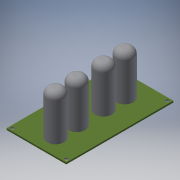
# Autodesk Inventor part: PCB
Saved by Autodesk Inventor 2017 (Build 210142000, 142)
## iProperties
Created: 2018-01-14
Part Number: PCB
Material: Generic
Document SubType Name: Modeling
Designer: Mitch
Density: 1 g/cm^3
Appearance: Default
Author: Mitch
Autodesk Inventor part; units mm, degrees
ref_plane "YZ Plane" through (0, 0, 0) normal (1, 0, 0) x (0, 1, 0)
ref_plane "XZ Plane" through (0, 0, 0) normal (0, 1, 0) x (-1, 0, 0)
ref_plane "XY Plane" through (0, 0, 0) normal (0, 0, 1) x (1, 0, 0)
sketch "Sketch3" plane through (0, 0, 0) normal (0, 1, 0) x (-1, 0, 0)
  line L0 (0, 0) -> (62.23, 0)
  line L1 (62.23, 0) -> (62.23, -111.76)
  line L2 (62.23, -111.76) -> (0, -111.76)
  line L3 (0, -111.76) -> (0, 0)
  dimension "d53" = 62.23
  dimension "d54" = 111.76
  constraints: 8 end point, 2 parallel, 1 horizontal, 1 perpendicular
  measures "d53" distance of L1.end L2.end
  measures "d54" distance of L0.end L1.end
extrude "Extrusion4" add sketch "Sketch3" along normal blind 1.5748
sketch "Sketch4" plane through (0, 1.5748, 0) normal (0, 1, 0) x (1, 0, 0)
  line L0 (-62.23, 0) -> (0, 0) projected
  line L1 (0, 0) -> (0, 111.76) projected
  line L2 (0, 111.76) -> (-62.23, 111.76) projected
  line L3 (-62.23, 111.76) -> (-62.23, 0) projected
  circle A0 centre (-59.055, 3.175) radius 1.7266
  circle A1 centre (-59.055, 108.585) radius 1.7266
  circle A2 centre (-3.175, 108.585) radius 1.7266
  circle A3 centre (-3.175, 3.175) radius 1.7266
  dimension "d57" = 3.4531
  dimension "d58" = 3.4531
  dimension "d59" = 3.4531
  dimension "d60" = 3.4531
  dimension "d61" = 3.175
  dimension "d62" = 3.175
  dimension "d63" = 3.175
  dimension "d64" = 3.175
  dimension "d65" = 3.175
  dimension "d66" = 3.175
  dimension "d67" = 3.175
  dimension "d68" = 3.175
  constraints: 4 centre point
  measures "d57" diameter of A0
  measures "d58" diameter of A1
  measures "d59" diameter of A2
  measures "d60" diameter of A3
  measures "d61" distance from line of L0 A0.centre
  measures "d62" distance from line of L3 A0.centre
  measures "d63" distance from line of L2 A1.centre
  measures "d64" distance from line of L3 A1.centre
  measures "d65" distance from line of A2.centre L2
  measures "d66" distance from line of L1 A2.centre
  measures "d67" distance from line of L1 A3.centre
  measures "d68" distance from line of L0 A3.centre
extrude "Extrusion5" cut sketch "Sketch4" against normal blind 2.54 contours A0 | A1 | A2 | A3
sketch "Sketch5" plane through (0, 1.5748, 0) normal (0, 1, 0) x (1, 0, 0)
  circle A0 centre (-28.448, 17.272) radius 8.9535
  circle A1 centre (-28.448, 39.37) radius 8.9535
  circle A2 centre (-28.448, 67.31) radius 8.9535
  circle A3 centre (-28.448, 89.408) radius 8.9535
  line L0 (-62.23, 0) -> (0, 0) projected
  line L1 (0, 0) -> (0, 111.76) projected
  line L2 (-62.23, 111.76) -> (-62.23, 0) projected
  dimension "d71" = 17.907
  dimension "d72" = 17.907
  dimension "d73" = 17.907
  dimension "d74" = 17.907
  dimension "d75" = 17.272
  dimension "d78" = 22.098
  dimension "d80" = 27.94
  dimension "d82" = 22.098
  dimension "d86" = 33.782
  constraints: 4 centre point
  measures "d71" diameter of A0
  measures "d72" diameter of A1
  measures "d73" diameter of A2
  measures "d74" diameter of A3
  measures "d75" distance from line of L0 A0.centre
  measures "d78" distance of A0.centre A1.centre
  measures "d80" distance of A1.centre A2.centre
  measures "d82" distance of A2.centre A3.centre
  measures "d86" distance from line of A0.centre L2
extrude "Extrusion6" add sketch "Sketch5" along normal blind 45.72
fillet "Fillet2" radius 6.35 4 edges at (-37.4015, 47.2948, -17.272) (-37.4015, 47.2948, -39.37) (-37.4015, 47.2948, -67.31) (-37.4015, 47.2948, -89.408)
sketch "Sketch6" plane through (0, 1.5748, 0) normal (0, 1, 0) x (1, 0, 0)
  line L0 (-62.23, 111.76) -> (-62.23, 0) projected
  line L1 (-62.23, 0) -> (-62.23, 42.672)
  line L2 (-62.23, 42.672) -> (-60.198, 42.672)
  line L3 (-60.198, 42.672) -> (-60.198, 65.532)
  line L4 (-60.198, 65.532) -> (-62.23, 65.532)
  line L5 (-62.23, 42.672) -> (-62.23, 65.532)
  point P0 (0, 0)
  dimension "d87" = 42.672
  dimension "d88" = 2.032
  dimension "d89" = 22.86
  constraints: 10 end point, 3 perpendicular, 2 point on line, 1 horizontal
  measures "d87" distance of L0.end L1.end
  measures "d88" distance of L1.end L2.end
  measures "d89" distance of L2.end L3.end
extrude "Extrusion7" cut sketch "Sketch6" against normal blind 45.72
body "Solid2"
